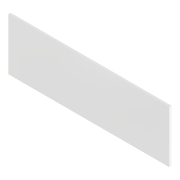
# Autodesk Inventor part: 00_Sample
Saved by Autodesk Inventor 2022.5 (Build 265521000, 521)
## iProperties
Created: 2023-11-08
Part Number: 00_Sample
Material: Generisch
Document SubType Name: Modeling
Designer: diederichbenedict
Density: 1 g/cm^3
Appearance: Polycarbonat - klar
Author: diederichbenedict
Autodesk Inventor part; units mm, degrees
ref_plane "YZ Plane" through (0, 0, 0) normal (1, 0, 0) x (0, 1, 0)
ref_plane "XZ Plane" through (0, 0, 0) normal (0, 1, 0) x (-1, 0, 0)
ref_plane "XY Plane" through (0, 0, 0) normal (0, 0, 1) x (1, 0, 0)
sketch "Skizze1" plane through (0, 0, 0) normal (0, 0, 1) x (1, 0, 0)
  line L0 (-37, 12) -> (37, 12)
  line L1 (37, 12) -> (37, -12)
  line L2 (37, -12) -> (-37, -12)
  line L3 (-37, -12) -> (-37, 12)
  line L4 (-37, 12) -> (37, -12) construction
  line L5 (37, 12) -> (-37, -12) construction
  line L6 (-37, 12) -> (37, 12) construction
  point P0 (0, 0)
  dimension "d0" = 74
  dimension "d1" = 0
  dimension "d2" = 24
  constraints: 14 end point, 2 horizontal, 2 midpoint, 2 parallel, 1 collinear, 1 perpendicular
  measures "d0" distance of L0.start L0.end
  measures "d1" distance between parallel lines of L0 L6
  measures "d2" distance of L0.end L1.end
extrude "Extrusion1" add sketch "Skizze1" along normal blind 1
